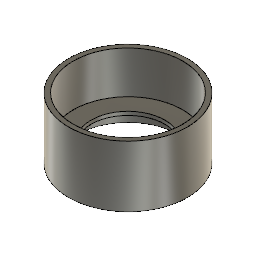
ME-eyeguard (Autodesk Fusion 360 design; units mm, degrees)
Autodesk Fusion 360 part; units mm, degrees
sketch "Sketch1" plane through (0, 0, 0) normal (0, 0, 1) x (1, 0, 0)
  circle A0 centre (0, 0) radius 20
  circle A1 centre (0, 0) radius 18.4
  circle A2 centre (0, 0) radius 12.4
  circle A3 centre (0, 0) radius 16.8
  dimension "d1" = 40
  dimension "d2" = -1.6
  dimension "d3" = -7.6
  dimension "d4" = -3.2
  constraint coincident A0.centre A1.centre
  measures "d1" diameter of A0
extrude "Extrude1" add sketch "Sketch1" against normal blind 6.4 contours A0 | A1
extrude "Extrude2" add sketch "Sketch1" against normal blind 1.2 contours A3
extrude "Extrude3" add sketch "Sketch1" along normal blind 9.2 contours A0
extrude "Extrude4" add 1 faces at (19.3922, -0.9936, 9.2) along direction (0, 0, 1) blind 5
named bodies: "Eye Guard"
